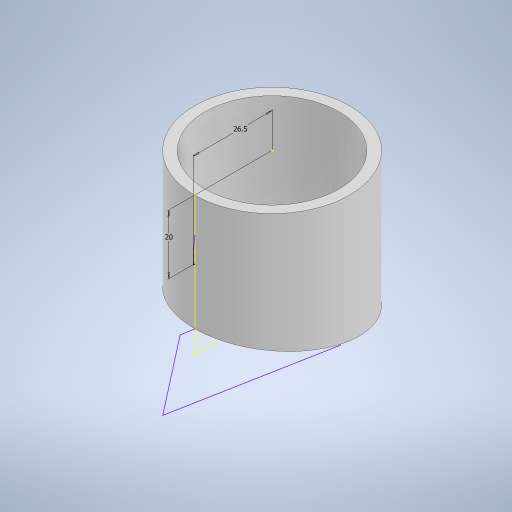
# Autodesk Inventor part: ElectricCarChargingPlugHolder2
Saved by Autodesk Inventor 2023 (Build 270158000, 158)
## iProperties
Created: 2023-08-16
Part Number: ElectricCarChargingPlugHolder2
Material: Generic
Document SubType Name: Modeling
Designer: lidang
Density: 1 g/cm^3
Appearance: Default
Author: lidang
Autodesk Inventor part; units mm, degrees
ref_plane "YZ Plane" through (0, 0, 0) normal (1, 0, 0) x (0, 1, 0)
ref_plane "XZ Plane" through (0, 0, 0) normal (0, 1, 0) x (-1, 0, 0)
ref_plane "XY Plane" through (0, 0, 0) normal (0, 0, 1) x (1, 0, 0)
sketch "Sketch1" plane through (0, 0, 0) normal (0, 0, 1) x (1, 0, 0)
  line L0 (0, 0) -> (-22.5, 0)
  line L1 (-22.5, 0) -> (-22.5, -36)
  line L2 (-22.5, -36) -> (0, -36)
  line L3 (0, -36) -> (0, 0)
  line L4 (-22.5, 0) -> (-26, 0)
  line L5 (0, -36) -> (0, -46)
  line L6 (0, -46) -> (-26, -46)
  line L7 (-26, 0) -> (-26, -46)
  dimension "d2" = 22.5
  dimension "d3" = 36
  dimension "d4" = 3.5
  dimension "d5" = 10
  constraints: 16 end point, 5 perpendicular, 1 horizontal, 1 point on line, 1 vertical
  measures "d2" distance of L0.start L0.end
  measures "d3" distance of L0.end L1.end
  measures "d4" distance of L0.end L4.end
  measures "d5" distance of L2.end L5.end
revolve "Revolution1" add sketch "Sketch1" angle 360 about axis through (0, -36, 0) along (0, 1, 0) contours L1 L2 L5 L6 L7 L4
sketch "Sketch2" plane through (0, 0, 0) normal (1, 0, 0) x (0, 1, 0)
  line L0 (-36, -22.5) -> (-36, 22.5) projected
  line L1 (-38.2014, 30.963) -> (-46, -26)
  line L2 (-46, -26) -> (0, -26) projected
  line L3 (-68.1118, -22.9728) -> (-58.6737, 36.8195)
  line L4 (-58.6737, 36.8195) -> (-38.2014, 30.963)
  line L5 (-46, -26) -> (-46, 26) projected
  line L6 (-68.1118, -22.9728) -> (-46, -26)
  line L7 (-2.125, 25.0163) -> (-16.5565, 26.5)
  line L8 (-16.5565, 26.5) -> (-20, 26.5)
  line L9 (-46, 26) -> (0, 26) projected
  line L10 (-20, 26.5) -> (-20, 23.9468)
  line L11 (-46, 26) -> (0, 26) projected
  line L12 (-20, 23.9468) -> (-2.125, 25.0163)
  line L13 (-20, 23.9468) -> (-20, 26)
  line L14 (-46, 26) -> (0, 26) projected
  line L15 (-46, 26) -> (0, 26) projected
  line L16 (-29.3452, 26) -> (-29.2838, 24.9734)
  line L17 (-29.2838, 24.9734) -> (-20, 23.9468)
  point P0 (0, 0)
  dimension "d11" = 20
  dimension "d12" = 26.5
  constraints: 22 end point, 3 perpendicular, 3 point on line, 1 parallel, 2 other
  measures "d11" distance from line of point (0, 0) L10
  measures "d12" distance from line of point (0, 0) L8
extrude "Extrusion1" cut sketch "Sketch2" along normal through all both and the other way through all contours L1 L9 L5 L6 L3 L4 | L1 L5 L9
body "Solid1"
